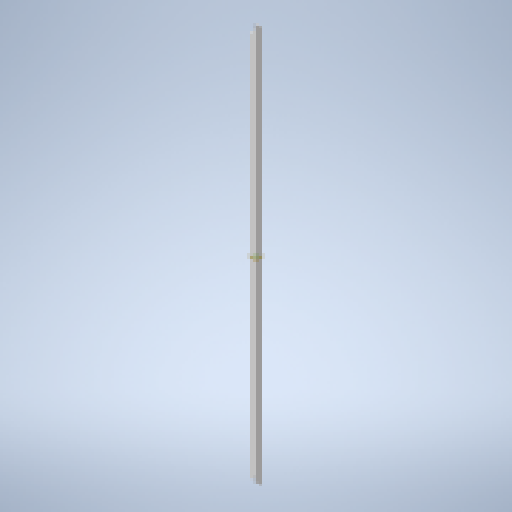
# Autodesk Inventor part: Perfil
Saved by Autodesk Inventor 2024 (Build 280153000, 153)
## iProperties
Created: 2023-07-24
Part Number: Perfil
Material: Genérico
Document SubType Name: Modeling
Designer: sergi
Density: 1 g/cm^3
Appearance: Valor por defecto
Author: sergi
Autodesk Inventor part; units mm, degrees
ref_plane "YZ Plane" through (0, 0, 0) normal (1, 0, 0) x (0, 1, 0)
ref_plane "XZ Plane" through (0, 0, 0) normal (0, 1, 0) x (-1, 0, 0)
ref_plane "XY Plane" through (0, 0, 0) normal (0, 0, 1) x (1, 0, 0)
sketch "Boceto1" plane through (0, 0, 0) normal (0, 1, 0) x (-1, 0, 0)
  line L0 (0, 0) -> (1.1, 0)
  line L1 (1.1, 0) -> (1.1, -10.9)
  line L2 (0.6, -11.4) -> (-10.3, -11.4)
  line L3 (-10.3, -11.4) -> (-10.3, -10.3)
  line L4 (-10.3, -10.3) -> (-0.5, -10.3)
  line L5 (0, -9.8) -> (0, 0)
  arc A0 (-0.5, -10.3) -> (0, -9.8) centre (-0.5, -9.8) ccw
  arc A1 (0.6, -11.4) -> (1.1, -10.9) centre (0.6, -10.9) ccw
  point P0 (1.1, -11.4)
  dimension "d0" = 1.1
  dimension "d1" = 11.4
  dimension "d2" = 11.4
  dimension "d3" = 1.1
  dimension "d4" = 0.5
  constraints: 12 end point, 5 perpendicular, 4 point on circle, 4 tangent, 2 centre point, 2 point on line, 1 equal radius, 1 horizontal
  measures "d0" distance of L0.start L0.end
  measures "d1" distance of L0.end point (1.1, -11.4)
  measures "d2" distance of point (1.1, -11.4) L2.end
  measures "d3" distance of L2.end L3.end
  measures "d4" radius of A0
extrude "Extrusión1" add sketch "Boceto1" along normal blind 750
ref_plane "Plano de trabajo1" through (0, 375, 0) normal (0, -1, 0) x (1, 0, 0)
